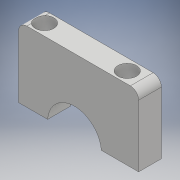
# Autodesk Inventor part: CarroXY - HotendFrente
Saved by Autodesk Inventor 2017 (Build 210142000, 142)
## iProperties
Created: 2020-09-05
Part Number: CarroXY - HotendFrente
Material: Generic
Document SubType Name: Modeling
Designer: ale
Density: 1 g/cm^3
Appearance: Default
Author: ale
Autodesk Inventor part; units mm, degrees
ref_plane "YZ Plane" through (0, 0, 0) normal (1, 0, 0) x (0, 1, 0)
ref_plane "XZ Plane" through (0, 0, 0) normal (0, 1, 0) x (-1, 0, 0)
ref_plane "XY Plane" through (0, 0, 0) normal (0, 0, 1) x (1, 0, 0)
sketch "Sketch1" plane through (0, 0, 0) normal (0, 0, 1) x (1, 0, 0)
  line L0 (-14.5, 2.75) -> (14.5, 2.75)
  line L1 (14.5, 2.75) -> (14.5, -2.75)
  line L2 (14.5, -2.75) -> (-14.5, -2.75)
  line L3 (-14.5, -2.75) -> (-14.5, 2.75)
  line L4 (-14.5, 2.75) -> (14.5, -2.75) construction
  line L5 (14.5, 2.75) -> (-14.5, -2.75) construction
  point P0 (0, 0)
  dimension "d0" = 29
  dimension "d1" = 5.5
  constraints: 12 end point, 2 midpoint, 2 parallel, 1 horizontal, 1 perpendicular
  measures "d0" distance of L1.end L2.end
  measures "d1" distance of L0.end L1.end
extrude "Extrusion1" add sketch "Sketch1" along normal blind 17
sketch "Sketch2" plane through (-14.5, 2.75, 0) normal (0, 1, 0) x (1, 0, 0)
  circle A0 centre (13.5, 0.5) radius 6.5
  line L0 (0, 0) -> (0, -17) projected
  line L1 (29, -17) -> (0, -17) projected
  point P0 (19.9809, 0.0015)
  point P1 (7.0191, 0.0015)
  dimension "d5" = 13
  dimension "d6" = 13.5
  dimension "d10" = 17.5
  constraints: 2 point on circle, 1 centre point
  measures "d5" diameter of A0
  measures "d6" distance from line of A0.centre L0
  measures "d10" distance from line of A0.centre L1
extrude "Extrusion2" cut sketch "Sketch2" against normal through all
sketch "Sketch3" plane through (0, 0, 0) normal (0, 0, -1) x (-1, 0, 0)
  circle A0 centre (11, 0) radius 2.25
  line L0 (7.4807, -2.75) -> (14.5, -2.75) projected
  line L1 (14.5, -2.75) -> (14.5, 2.75) projected
  circle A1 centre (-9, 0) radius 2.25
  line L2 (-14.5, -2.75) -> (-5.4807, -2.75) projected
  point P0 (0, 0)
  dimension "d11" = 4.5
  dimension "d12" = 2.75
  dimension "d13" = 3.5
  dimension "d14" = 4.5
  dimension "d15" = 20
  dimension "d16" = 2.75
  constraints: 2 centre point
  measures "d11" diameter of A0
  measures "d12" distance from line of A0.centre L0
  measures "d13" distance from line of L1 A0.centre
  measures "d14" diameter of A1
  measures "d15" distance of A1.centre A0.centre
  measures "d16" distance from line of L2 A1.centre
hole "Hole1" at (9, 0, 0) at (-11, 0, 0) direction (0, 0, 1) diameter 4.5 end through all
fillet "Fillet1" radius 2 2 edges at (-14.5, 0, 17) (14.5, 0, 17)
body "Solid1"
